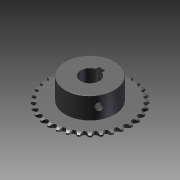
# Autodesk Inventor part: SP25B32-N-15_b
Saved by Autodesk Inventor 2011 SP1 (Build 150282100, 282)
## iProperties
Created: 2016-11-23
Part Number: SP25B32-N-15_b
Catalog Web Link: www.cadenas.de
Description: SP25B, SSP25B_base-Sprocket 25B
Vendor: MISUMI
Document SubType Name: Modeling
Designer: psAdmin
Manufacturer: MISUMI
Mass: 26.4316 g
Surface Area: 103.47 cm^2
Volume: 26.4316 cm^3
Density: 1 g/cm^3
Category: PARTsolutions
Company: MISUMI
Title: SP25B32-N-15
Author: Cadenas PARTsolutions
Comments: Sprocket 25B
PSOL_IDENT_0: {$CADENAS_DATA\23d-libs\misumi\metric\55_chains_sprockets\sp25b\sp25b.prj},191 {VTYP=3D},{NB=SP25B32
PSOL_IDENT_1: -N-15_b},{LINA=SP25B32-N-15},{NN=SP25B, SSP25B_base},{DATE=17.06.2016 05:56:25},{GEOMDATE=06.03.2014
PSOL_IDENT_2: 01:18:00},{VERSION=},{LINEID=140},{LINESUBID=-1},{WBVAR=MAT,SPEC,D}  {NB=SP25B32-N-15_b},{LINA=SP25
PSOL_IDENT_3: B32-N-15},{KT=DUMMY},{PN=SP25B32-N-15},{TYPE=SP25B},{MAT=1},{MATA='1','1045 Carbon Steel Equivalent'
PSOL_IDENT_4: ,'2','304 Stainless Steel Equivalent'},{AC=Set Screw},{NT=32},{SPEC=N},{D=15},{DA1='15','15','16','1
PSOL_IDENT_5: 6','20','20'},{DA2='12','12','15','15'},{DPP=64.78},{DOO=68},{H=40},{L=20},{LL=8},{M=6},{BBTT=5x2.3}
PSOL_IDENT_6: ,{COS=4.917},{BB=5},{TT=2.3},{T=2.800},{DA='15','15','16','16','20','20'},{D1=15},{DA3='10','10'},{D
PSOL_IDENT_7: A4='10','10'},{DRR=3.3},{SSM=6.000},{SSL=6.000}
NN: SP25B, SSP25B_base
NT: 32
NB: SP25B32-N-15_b
NBSYN: $PN._b
LINA: SP25B32-N-15
PN: SP25B32-N-15
MAT: 1045 Carbon Steel Equivalent
AC: Set Screw
SPEC: New JIS Key Groove Hole Tapped
D: 15
DPP: 64.78
DOO: 68
H: 40
L: 20
LL: 8
M: 6
BBTT: 5x2.3
SUPPLIER: MISUMI
ARTICLENO: SP25B32-N-15_b
BOMINFO: SP25B32-N-15
CREATOR: CADENAS GmbH
Autodesk Inventor part; units mm, degrees
sketch "Sketch_1" plane through (0, 0, 0) normal (1, 0, 0) x (0, 1, 0)
  line L0 (0, 0) -> (0, 1.4)
  line L1 (7.5, 20) -> (7.5, 0)
  line L2 (7.5, 0) -> (30.825225, 0)
  arc A0 (30.825225, 0) -> (34, 0.850678) centre (30.825225, 6.34955) ccw
  line L3 (34, 0.850678) -> (34, 1.949322)
  arc A1 (34, 1.949322) -> (30.825225, 2.8) centre (30.825225, -3.54955) ccw
  line L4 (30.825225, 2.8) -> (20, 2.8)
  line L5 (20, 2.8) -> (20, 19.8)
  line L6 (20, 19.8) -> (19.8, 20)
  line L7 (19.8, 20) -> (7.5, 20)
  constraints: 16 end point, 4 point on circle, 2 centre point
revolve "Revolution1" add sketch "Sketch_1" angle 360 about axis through (0, 0, 0) along (0, 0, -1)
sketch "Sketch_2" plane through (0, 0, 0) normal (0, 0, 1) x (1, 0, 0)
  circle A0 centre (0, 0) radius 64.78
  line L0 (-34, 0.762388) -> (-34, -0.762388)
  line L1 (-34, -0.762388) -> (-31.661667, -1.62723)
  arc A1 (-31.370754, -4.580922) -> (-31.661667, -1.62723) centre (-32.234033, -3.174775) ccw
  line L2 (-31.370754, -4.580922) -> (-33.495434, -5.885332)
  line L3 (-33.495434, -5.885332) -> (-33.197965, -7.380809)
  line L4 (-33.197965, -7.380809) -> (-30.73584, -7.772848)
  arc A2 (-29.87428, -10.613031) -> (-30.73584, -7.772848) centre (-30.995297, -9.402321) ccw
  line L5 (-29.87428, -10.613031) -> (-31.703657, -12.306882)
  line L6 (-31.703657, -12.306882) -> (-31.120151, -13.715591)
  line L7 (-31.120151, -13.715591) -> (-28.628852, -13.61976)
  arc A3 (-27.229755, -16.237288) -> (-28.628852, -13.61976) centre (-28.56543, -15.26854) ccw
  line L8 (-27.229755, -16.237288) -> (-28.693527, -18.255486)
  line L9 (-28.693527, -18.255486) -> (-27.846407, -19.52329)
  line L10 (-27.846407, -19.52329) -> (-25.421674, -18.943272)
  arc A4 (-23.538805, -21.237554) -> (-25.421674, -18.943272) centre (-25.037809, -20.547998) ccw
  line L11 (-23.538805, -21.237554) -> (-24.58072, -23.502541)
  line L12 (-24.58072, -23.502541) -> (-23.502541, -24.58072)
  line L13 (-23.502541, -24.58072) -> (-21.237554, -23.538805)
  arc A5 (-18.943272, -25.421674) -> (-21.237554, -23.538805) centre (-20.547998, -25.037809) ccw
  line L14 (-18.943272, -25.421674) -> (-19.52329, -27.846407)
  line L15 (-19.52329, -27.846407) -> (-18.255486, -28.693527)
  line L16 (-18.255486, -28.693527) -> (-16.237288, -27.229755)
  arc A6 (-13.61976, -28.628852) -> (-16.237288, -27.229755) centre (-15.26854, -28.56543) ccw
  line L17 (-13.61976, -28.628852) -> (-13.715591, -31.120151)
  line L18 (-13.715591, -31.120151) -> (-12.306882, -31.703657)
  line L19 (-12.306882, -31.703657) -> (-10.613031, -29.87428)
  arc A7 (-7.772848, -30.73584) -> (-10.613031, -29.87428) centre (-9.402321, -30.995297) ccw
  line L20 (-7.772848, -30.73584) -> (-7.380809, -33.197965)
  line L21 (-7.380809, -33.197965) -> (-5.885332, -33.495434)
  line L22 (-5.885332, -33.495434) -> (-4.580922, -31.370754)
  arc A8 (-1.62723, -31.661667) -> (-4.580922, -31.370754) centre (-3.174775, -32.234033) ccw
  line L23 (-1.62723, -31.661667) -> (-0.762388, -34)
  line L24 (-0.762388, -34) -> (0.762388, -34)
  line L25 (0.762388, -34) -> (1.62723, -31.661667)
  arc A9 (4.580922, -31.370754) -> (1.62723, -31.661667) centre (3.174775, -32.234033) ccw
  line L26 (4.580922, -31.370754) -> (5.885332, -33.495434)
  line L27 (5.885332, -33.495434) -> (7.380809, -33.197965)
  line L28 (7.380809, -33.197965) -> (7.772848, -30.73584)
  arc A10 (10.613031, -29.87428) -> (7.772848, -30.73584) centre (9.402321, -30.995297) ccw
  line L29 (10.613031, -29.87428) -> (12.306882, -31.703657)
  line L30 (12.306882, -31.703657) -> (13.715591, -31.120151)
  line L31 (13.715591, -31.120151) -> (13.61976, -28.628852)
  arc A11 (16.237288, -27.229755) -> (13.61976, -28.628852) centre (15.26854, -28.56543) ccw
  line L32 (16.237288, -27.229755) -> (18.255486, -28.693527)
  line L33 (18.255486, -28.693527) -> (19.52329, -27.846407)
  line L34 (19.52329, -27.846407) -> (18.943272, -25.421674)
  arc A12 (21.237554, -23.538805) -> (18.943272, -25.421674) centre (20.547998, -25.037809) ccw
  line L35 (21.237554, -23.538805) -> (23.502541, -24.58072)
  line L36 (23.502541, -24.58072) -> (24.58072, -23.502541)
  line L37 (24.58072, -23.502541) -> (23.538805, -21.237554)
  arc A13 (25.421674, -18.943272) -> (23.538805, -21.237554) centre (25.037809, -20.547998) ccw
  line L38 (25.421674, -18.943272) -> (27.846407, -19.52329)
  line L39 (27.846407, -19.52329) -> (28.693527, -18.255486)
  line L40 (28.693527, -18.255486) -> (27.229755, -16.237288)
  arc A14 (28.628852, -13.61976) -> (27.229755, -16.237288) centre (28.56543, -15.26854) ccw
  line L41 (28.628852, -13.61976) -> (31.120151, -13.715591)
  line L42 (31.120151, -13.715591) -> (31.703657, -12.306882)
  line L43 (31.703657, -12.306882) -> (29.87428, -10.613031)
  arc A15 (30.73584, -7.772848) -> (29.87428, -10.613031) centre (30.995297, -9.402321) ccw
  line L44 (30.73584, -7.772848) -> (33.197965, -7.380809)
  line L45 (33.197965, -7.380809) -> (33.495434, -5.885332)
  line L46 (33.495434, -5.885332) -> (31.370754, -4.580922)
  arc A16 (31.661667, -1.62723) -> (31.370754, -4.580922) centre (32.234033, -3.174775) ccw
  line L47 (31.661667, -1.62723) -> (34, -0.762388)
  line L48 (34, -0.762388) -> (34, 0.762388)
  line L49 (34, 0.762388) -> (31.661667, 1.62723)
  arc A17 (31.370754, 4.580922) -> (31.661667, 1.62723) centre (32.234033, 3.174775) ccw
  line L50 (31.370754, 4.580922) -> (33.495434, 5.885332)
  line L51 (33.495434, 5.885332) -> (33.197965, 7.380809)
  line L52 (33.197965, 7.380809) -> (30.73584, 7.772848)
  arc A18 (29.87428, 10.613031) -> (30.73584, 7.772848) centre (30.995297, 9.402321) ccw
  line L53 (29.87428, 10.613031) -> (31.703657, 12.306882)
  line L54 (31.703657, 12.306882) -> (31.120151, 13.715591)
  line L55 (31.120151, 13.715591) -> (28.628852, 13.61976)
  arc A19 (27.229755, 16.237288) -> (28.628852, 13.61976) centre (28.56543, 15.26854) ccw
  line L56 (27.229755, 16.237288) -> (28.693527, 18.255486)
  line L57 (28.693527, 18.255486) -> (27.846407, 19.52329)
  line L58 (27.846407, 19.52329) -> (25.421674, 18.943272)
  arc A20 (23.538805, 21.237554) -> (25.421674, 18.943272) centre (25.037809, 20.547998) ccw
  line L59 (23.538805, 21.237554) -> (24.58072, 23.502541)
  line L60 (24.58072, 23.502541) -> (23.502541, 24.58072)
  line L61 (23.502541, 24.58072) -> (21.237554, 23.538805)
  arc A21 (18.943272, 25.421674) -> (21.237554, 23.538805) centre (20.547998, 25.037809) ccw
  line L62 (18.943272, 25.421674) -> (19.52329, 27.846407)
  line L63 (19.52329, 27.846407) -> (18.255486, 28.693527)
  line L64 (18.255486, 28.693527) -> (16.237288, 27.229755)
  arc A22 (13.61976, 28.628852) -> (16.237288, 27.229755) centre (15.26854, 28.56543) ccw
  line L65 (13.61976, 28.628852) -> (13.715591, 31.120151)
  line L66 (13.715591, 31.120151) -> (12.306882, 31.703657)
  line L67 (12.306882, 31.703657) -> (10.613031, 29.87428)
  arc A23 (7.772848, 30.73584) -> (10.613031, 29.87428) centre (9.402321, 30.995297) ccw
  line L68 (7.772848, 30.73584) -> (7.380809, 33.197965)
  line L69 (7.380809, 33.197965) -> (5.885332, 33.495434)
  line L70 (5.885332, 33.495434) -> (4.580922, 31.370754)
  arc A24 (1.62723, 31.661667) -> (4.580922, 31.370754) centre (3.174775, 32.234033) ccw
  line L71 (1.62723, 31.661667) -> (0.762388, 34)
  line L72 (0.762388, 34) -> (-0.762388, 34)
  line L73 (-0.762388, 34) -> (-1.62723, 31.661667)
  arc A25 (-4.580922, 31.370754) -> (-1.62723, 31.661667) centre (-3.174775, 32.234033) ccw
  line L74 (-4.580922, 31.370754) -> (-5.885332, 33.495434)
  line L75 (-5.885332, 33.495434) -> (-7.380809, 33.197965)
  line L76 (-7.380809, 33.197965) -> (-7.772848, 30.73584)
  arc A26 (-10.613031, 29.87428) -> (-7.772848, 30.73584) centre (-9.402321, 30.995297) ccw
  line L77 (-10.613031, 29.87428) -> (-12.306882, 31.703657)
  line L78 (-12.306882, 31.703657) -> (-13.715591, 31.120151)
  line L79 (-13.715591, 31.120151) -> (-13.61976, 28.628852)
  arc A27 (-16.237288, 27.229755) -> (-13.61976, 28.628852) centre (-15.26854, 28.56543) ccw
  line L80 (-16.237288, 27.229755) -> (-18.255486, 28.693527)
  line L81 (-18.255486, 28.693527) -> (-19.52329, 27.846407)
  line L82 (-19.52329, 27.846407) -> (-18.943272, 25.421674)
  arc A28 (-21.237554, 23.538805) -> (-18.943272, 25.421674) centre (-20.547998, 25.037809) ccw
  line L83 (-21.237554, 23.538805) -> (-23.502541, 24.58072)
  line L84 (-23.502541, 24.58072) -> (-24.58072, 23.502541)
  line L85 (-24.58072, 23.502541) -> (-23.538805, 21.237554)
  arc A29 (-25.421674, 18.943272) -> (-23.538805, 21.237554) centre (-25.037809, 20.547998) ccw
  line L86 (-25.421674, 18.943272) -> (-27.846407, 19.52329)
  line L87 (-27.846407, 19.52329) -> (-28.693527, 18.255486)
  line L88 (-28.693527, 18.255486) -> (-27.229755, 16.237288)
  arc A30 (-28.628852, 13.61976) -> (-27.229755, 16.237288) centre (-28.56543, 15.26854) ccw
  line L89 (-28.628852, 13.61976) -> (-31.120151, 13.715591)
  line L90 (-31.120151, 13.715591) -> (-31.703657, 12.306882)
  line L91 (-31.703657, 12.306882) -> (-29.87428, 10.613031)
  arc A31 (-30.73584, 7.772848) -> (-29.87428, 10.613031) centre (-30.995297, 9.402321) ccw
  line L92 (-30.73584, 7.772848) -> (-33.197965, 7.380809)
  line L93 (-33.197965, 7.380809) -> (-33.495434, 5.885332)
  line L94 (-33.495434, 5.885332) -> (-31.370754, 4.580922)
  arc A32 (-31.661667, 1.62723) -> (-31.370754, 4.580922) centre (-32.234033, 3.174775) ccw
  line L95 (-31.661667, 1.62723) -> (-34, 0.762388)
  constraints: 192 end point, 64 point on circle, 33 centre point
extrude "Extrusion1" cut sketch "Sketch_2" along normal blind 2.8
sketch "Sketch_3" plane through (0, 0, 12) normal (0, 0, 1) x (1, 0, 0)
  line L0 (0, 20) -> (0, 7)
  line L1 (0, 7) -> (-2.4585, 7)
  line L2 (-2.4585, 7) -> (-2.4585, 19.4585)
  line L3 (-2.4585, 19.4585) -> (-3, 20)
  line L4 (-3, 20) -> (0, 20)
  line L5 (0, 20) -> (0, 7)
  constraints: 12 end point
revolve "Revolution2" cut sketch "Sketch_3" angle 360 about axis through (0, 20, 12) along (0, 1, 0)
thread "Thread1" size "M6x1" class "6H" standard "ISO Metric profile" length 9.6585
sketch "Sketch_7" plane through (0, 0, 12) normal (0, 0, 1) x (1, 0, 0)
  line L0 (17.320508, -10) -> (0, 0)
  line L1 (0, 0) -> (1.22925, 2.129123)
  line L2 (1.22925, 2.129123) -> (18.080805, -7.600127)
  line L3 (18.080805, -7.600127) -> (18.820508, -7.401924)
  line L4 (18.820508, -7.401924) -> (17.320508, -10)
  line L5 (17.320508, -10) -> (0, 0)
  constraints: 12 end point
revolve "Revolution3" cut sketch "Sketch_7" angle 360 about axis through (17.320508, -10, 12) along (0.8660254, -0.5, 0)
thread "Thread2" size "M6x1" class "6H" standard "ISO Metric profile" length 11.9585
sketch "Sketch_5" plane through (0, 0, 0) normal (0, 0, 1) x (1, 0, 0)
  line L0 (-2.5, 0) -> (2.5, 0)
  line L1 (2.5, 0) -> (2.5, 9.8)
  line L2 (2.5, 9.8) -> (-2.5, 9.8)
  line L3 (-2.5, 9.8) -> (-2.5, 0)
  constraints: 8 end point
extrude "Extrusion2" cut sketch "Sketch_5" along normal blind 20
ref_plane "to_screw_1_XY" through (0, 9.8, 12) normal (0, 1, 0) x (1, 0, 0)
ref_plane "to_screw_1_YZ" through (0, 9.8, 12) normal (1, 0, 0) x (0, 0, -1)
ref_plane "to_screw_1_ZX" through (0, 9.8, 12) normal (0, 0, -1) x (0, 1, 0)
ref_plane "to_screw_2_XY" through (6.495191, -3.75, 12) normal (0.8660254, -0.5, 0) x (-0.5, -0.8660254, 0)
ref_plane "to_screw_2_YZ" through (6.495191, -3.75, 12) normal (-0.5, -0.8660254, 0) x (0, 0, -1)
ref_plane "to_screw_2_ZX" through (6.495191, -3.75, 12) normal (0, 0, -1) x (0.8660254, -0.5, 0)
body "Solid1"
